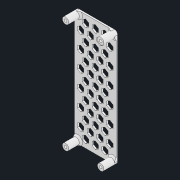
# Autodesk Inventor part: scara-base30
Saved by Autodesk Inventor 2022 (Build 260153000, 153)
## iProperties
Created: 2021-11-06
Part Number: scara-base30
Material: ABS プラスチック
Document SubType Name: Modeling
Designer: Yuta Kage
Density: 1.06 g/cm^3
Appearance: 滑らか - 白
Author: Yuta Kage
Autodesk Inventor part; units mm, degrees
ref_plane "YZ Plane" through (0, 0, 0) normal (1, 0, 0) x (0, 1, 0)
ref_plane "XZ Plane" through (0, 0, 0) normal (0, 1, 0) x (-1, 0, 0)
ref_plane "XY Plane" through (0, 0, 0) normal (0, 0, 1) x (1, 0, 0)
sketch "スケッチ1" plane through (0, 0, 0) normal (0, 0, 1) x (1, 0, 0)
  line L0 (-25.75, -71.75) -> (25.75, -71.75)
  line L1 (25.75, -71.75) -> (25.75, 71.75)
  line L2 (25.75, 71.75) -> (-25.75, 71.75)
  line L3 (-25.75, 71.75) -> (-25.75, -71.75)
  point P0 (0, 0)
  dimension "d0" = 143.5
  dimension "d1" = 51.5
  dimension "d2" = 71.75
  dimension "d3" = 25.75
  constraints: 8 end point, 2 parallel, 1 horizontal, 1 perpendicular
  measures "d0" distance of L2.end L0.start
  measures "d1" distance of L1.end L2.end
  measures "d2" distance from line of point (0, 0) L2
  measures "d3" distance from line of point (0, 0) L3
extrude "押し出し1" add sketch "スケッチ1" along normal blind 2
sketch "スケッチ2" plane through (0, 0, 2) normal (0, 0, 1) x (1, 0, 0)
  line L0 (-12, -57.735) -> (-8, -60.0444)
  line L1 (-8, -60.0444) -> (-8, -64.6632)
  line L2 (-8, -64.6632) -> (-12, -66.9726)
  line L3 (-12, -66.9726) -> (-16, -64.6632)
  line L4 (-16, -64.6632) -> (-16, -60.0444)
  line L5 (-16, -60.0444) -> (-12, -57.735)
  line L6 (-18, -47.3427) -> (-14, -49.6521)
  line L7 (-14, -49.6521) -> (-14, -54.2709)
  line L8 (-14, -54.2709) -> (-18, -56.5803)
  line L9 (-18, -56.5803) -> (-22, -54.2709)
  line L10 (-22, -54.2709) -> (-22, -49.6521)
  line L11 (-22, -49.6521) -> (-18, -47.3427)
  line L12 (-25.75, 71.75) -> (-25.75, -71.75) construction
  line L13 (-25.75, -71.75) -> (25.75, -71.75) projected
  line L14 (-37.6, 0) -> (38.35, 0) construction
  line L15 (0, -104.0432) -> (0, 115.0089) construction
  line L16 (-18, -26.5581) -> (-14, -28.8675)
  line L17 (-22, -28.8675) -> (-18, -26.5581)
  line L18 (-14, -28.8675) -> (-14, -33.4863)
  line L19 (-22, -33.4863) -> (-22, -28.8675)
  line L20 (-14, -33.4863) -> (-18, -35.7957)
  line L21 (-18, -35.7957) -> (-22, -33.4863)
  line L22 (-12, -36.9504) -> (-8, -39.2598)
  line L23 (-16, -39.2598) -> (-12, -36.9504)
  line L24 (-8, -39.2598) -> (-8, -43.8786)
  line L25 (-16, -43.8786) -> (-16, -39.2598)
  line L26 (-8, -43.8786) -> (-12, -46.188)
  line L27 (-12, -46.188) -> (-16, -43.8786)
  line L28 (-6, -47.3427) -> (-2, -49.6521)
  line L29 (-10, -49.6521) -> (-6, -47.3427)
  line L30 (-2, -49.6521) -> (-2, -54.2709)
  line L31 (-10, -54.2709) -> (-10, -49.6521)
  line L32 (-2, -54.2709) -> (-6, -56.5803)
  line L33 (-6, -56.5803) -> (-10, -54.2709)
  line L34 (0, -57.735) -> (4, -60.0444)
  line L35 (-4, -60.0444) -> (0, -57.735)
  line L36 (4, -60.0444) -> (4, -64.6632)
  line L37 (-4, -64.6632) -> (-4, -60.0444)
  line L38 (4, -64.6632) -> (0, -66.9726)
  line L39 (0, -66.9726) -> (-4, -64.6632)
  line L40 (-6, -26.5581) -> (-2, -28.8675)
  line L41 (-10, -28.8675) -> (-6, -26.5581)
  line L42 (-2, -28.8675) -> (-2, -33.4863)
  line L43 (-10, -33.4863) -> (-10, -28.8675)
  line L44 (-2, -33.4863) -> (-6, -35.7957)
  line L45 (-6, -35.7957) -> (-10, -33.4863)
  line L46 (0, -36.9504) -> (4, -39.2598)
  line L47 (-4, -39.2598) -> (0, -36.9504)
  line L48 (4, -39.2598) -> (4, -43.8786)
  line L49 (-4, -43.8786) -> (-4, -39.2598)
  line L50 (4, -43.8786) -> (0, -46.188)
  line L51 (0, -46.188) -> (-4, -43.8786)
  line L52 (-18, -5.7735) -> (-14, -8.0829)
  line L53 (-22, -8.0829) -> (-18, -5.7735)
  line L54 (-14, -8.0829) -> (-14, -12.7017)
  line L55 (-22, -12.7017) -> (-22, -8.0829)
  line L56 (-14, -12.7017) -> (-18, -15.0111)
  line L57 (-18, -15.0111) -> (-22, -12.7017)
  line L58 (-12, -16.1658) -> (-8, -18.4752)
  line L59 (-16, -18.4752) -> (-12, -16.1658)
  line L60 (-8, -18.4752) -> (-8, -23.094)
  line L61 (-16, -23.094) -> (-16, -18.4752)
  line L62 (-8, -23.094) -> (-12, -25.4034)
  line L63 (-12, -25.4034) -> (-16, -23.094)
  line L64 (-6, -5.7735) -> (-2, -8.0829)
  line L65 (-10, -8.0829) -> (-6, -5.7735)
  line L66 (-2, -8.0829) -> (-2, -12.7017)
  line L67 (-10, -12.7017) -> (-10, -8.0829)
  line L68 (-2, -12.7017) -> (-6, -15.0111)
  line L69 (-6, -15.0111) -> (-10, -12.7017)
  line L70 (0, -16.1658) -> (4, -18.4752)
  line L71 (-4, -18.4752) -> (0, -16.1658)
  line L72 (4, -18.4752) -> (4, -23.094)
  line L73 (-4, -23.094) -> (-4, -18.4752)
  line L74 (4, -23.094) -> (0, -25.4034)
  line L75 (0, -25.4034) -> (-4, -23.094)
  line L76 (-18, 15.0111) -> (-14, 12.7017)
  line L77 (-22, 12.7017) -> (-18, 15.0111)
  line L78 (-14, 12.7017) -> (-14, 8.0829)
  line L79 (-22, 8.0829) -> (-22, 12.7017)
  line L80 (-14, 8.0829) -> (-18, 5.7735)
  line L81 (-18, 5.7735) -> (-22, 8.0829)
  line L82 (-12, 4.6188) -> (-8, 2.3094)
  line L83 (-16, 2.3094) -> (-12, 4.6188)
  line L84 (-8, 2.3094) -> (-8, -2.3094)
  line L85 (-16, -2.3094) -> (-16, 2.3094)
  line L86 (-8, -2.3094) -> (-12, -4.6188)
  line L87 (-12, -4.6188) -> (-16, -2.3094)
  line L88 (-6, 15.0111) -> (-2, 12.7017)
  line L89 (-10, 12.7017) -> (-6, 15.0111)
  line L90 (-2, 12.7017) -> (-2, 8.0829)
  line L91 (-10, 8.0829) -> (-10, 12.7017)
  line L92 (-2, 8.0829) -> (-6, 5.7735)
  line L93 (-6, 5.7735) -> (-10, 8.0829)
  line L94 (0, 4.6188) -> (4, 2.3094)
  line L95 (-4, 2.3094) -> (0, 4.6188)
  line L96 (4, 2.3094) -> (4, -2.3094)
  line L97 (-4, -2.3094) -> (-4, 2.3094)
  line L98 (4, -2.3094) -> (0, -4.6188)
  line L99 (0, -4.6188) -> (-4, -2.3094)
  line L100 (-18, 35.7957) -> (-14, 33.4863)
  line L101 (-22, 33.4863) -> (-18, 35.7957)
  line L102 (-14, 33.4863) -> (-14, 28.8675)
  line L103 (-22, 28.8675) -> (-22, 33.4863)
  line L104 (-14, 28.8675) -> (-18, 26.5581)
  line L105 (-18, 26.5581) -> (-22, 28.8675)
  line L106 (-12, 25.4034) -> (-8, 23.094)
  line L107 (-16, 23.094) -> (-12, 25.4034)
  line L108 (-8, 23.094) -> (-8, 18.4752)
  line L109 (-16, 18.4752) -> (-16, 23.094)
  line L110 (-8, 18.4752) -> (-12, 16.1658)
  line L111 (-12, 16.1658) -> (-16, 18.4752)
  line L112 (-6, 35.7957) -> (-2, 33.4863)
  line L113 (-10, 33.4863) -> (-6, 35.7957)
  line L114 (-2, 33.4863) -> (-2, 28.8675)
  line L115 (-10, 28.8675) -> (-10, 33.4863)
  line L116 (-2, 28.8675) -> (-6, 26.5581)
  line L117 (-6, 26.5581) -> (-10, 28.8675)
  line L118 (0, 25.4034) -> (4, 23.094)
  line L119 (-4, 23.094) -> (0, 25.4034)
  line L120 (4, 23.094) -> (4, 18.4752)
  line L121 (-4, 18.4752) -> (-4, 23.094)
  line L122 (4, 18.4752) -> (0, 16.1658)
  line L123 (0, 16.1658) -> (-4, 18.4752)
  line L124 (-18, 56.5803) -> (-14, 54.2709)
  line L125 (-22, 54.2709) -> (-18, 56.5803)
  line L126 (-14, 54.2709) -> (-14, 49.6521)
  line L127 (-22, 49.6521) -> (-22, 54.2709)
  line L128 (-14, 49.6521) -> (-18, 47.3427)
  line L129 (-18, 47.3427) -> (-22, 49.6521)
  line L130 (-12, 46.188) -> (-8, 43.8786)
  line L131 (-16, 43.8786) -> (-12, 46.188)
  line L132 (-8, 43.8786) -> (-8, 39.2598)
  line L133 (-16, 39.2598) -> (-16, 43.8786)
  line L134 (-8, 39.2598) -> (-12, 36.9504)
  line L135 (-12, 36.9504) -> (-16, 39.2598)
  line L136 (-6, 56.5803) -> (-2, 54.2709)
  line L137 (-10, 54.2709) -> (-6, 56.5803)
  line L138 (-2, 54.2709) -> (-2, 49.6521)
  line L139 (-10, 49.6521) -> (-10, 54.2709)
  line L140 (-2, 49.6521) -> (-6, 47.3427)
  line L141 (-6, 47.3427) -> (-10, 49.6521)
  line L142 (0, 46.188) -> (4, 43.8786)
  line L143 (-4, 43.8786) -> (0, 46.188)
  line L144 (4, 43.8786) -> (4, 39.2598)
  line L145 (-4, 39.2598) -> (-4, 43.8786)
  line L146 (4, 39.2598) -> (0, 36.9504)
  line L147 (0, 36.9504) -> (-4, 39.2598)
  line L148 (6, -47.3427) -> (10, -49.6521)
  line L149 (2, -49.6521) -> (6, -47.3427)
  line L150 (10, -49.6521) -> (10, -54.2709)
  line L151 (2, -54.2709) -> (2, -49.6521)
  line L152 (10, -54.2709) -> (6, -56.5803)
  line L153 (6, -56.5803) -> (2, -54.2709)
  line L154 (12, -57.735) -> (16, -60.0444)
  line L155 (8, -60.0444) -> (12, -57.735)
  line L156 (16, -60.0444) -> (16, -64.6632)
  line L157 (8, -64.6632) -> (8, -60.0444)
  line L158 (16, -64.6632) -> (12, -66.9726)
  line L159 (12, -66.9726) -> (8, -64.6632)
  line L160 (6, -26.5581) -> (10, -28.8675)
  line L161 (2, -28.8675) -> (6, -26.5581)
  line L162 (10, -28.8675) -> (10, -33.4863)
  line L163 (2, -33.4863) -> (2, -28.8675)
  line L164 (10, -33.4863) -> (6, -35.7957)
  line L165 (6, -35.7957) -> (2, -33.4863)
  line L166 (12, -36.9504) -> (16, -39.2598)
  line L167 (8, -39.2598) -> (12, -36.9504)
  line L168 (16, -39.2598) -> (16, -43.8786)
  line L169 (8, -43.8786) -> (8, -39.2598)
  line L170 (16, -43.8786) -> (12, -46.188)
  line L171 (12, -46.188) -> (8, -43.8786)
  line L172 (6, -5.7735) -> (10, -8.0829)
  line L173 (2, -8.0829) -> (6, -5.7735)
  line L174 (10, -8.0829) -> (10, -12.7017)
  line L175 (2, -12.7017) -> (2, -8.0829)
  line L176 (10, -12.7017) -> (6, -15.0111)
  line L177 (6, -15.0111) -> (2, -12.7017)
  line L178 (12, -16.1658) -> (16, -18.4752)
  line L179 (8, -18.4752) -> (12, -16.1658)
  line L180 (16, -18.4752) -> (16, -23.094)
  line L181 (8, -23.094) -> (8, -18.4752)
  line L182 (16, -23.094) -> (12, -25.4034)
  line L183 (12, -25.4034) -> (8, -23.094)
  line L184 (6, 15.0111) -> (10, 12.7017)
  line L185 (2, 12.7017) -> (6, 15.0111)
  line L186 (10, 12.7017) -> (10, 8.0829)
  line L187 (2, 8.0829) -> (2, 12.7017)
  line L188 (10, 8.0829) -> (6, 5.7735)
  line L189 (6, 5.7735) -> (2, 8.0829)
  line L190 (12, 4.6188) -> (16, 2.3094)
  line L191 (8, 2.3094) -> (12, 4.6188)
  line L192 (16, 2.3094) -> (16, -2.3094)
  line L193 (8, -2.3094) -> (8, 2.3094)
  line L194 (16, -2.3094) -> (12, -4.6188)
  line L195 (12, -4.6188) -> (8, -2.3094)
  line L196 (6, 35.7957) -> (10, 33.4863)
  line L197 (2, 33.4863) -> (6, 35.7957)
  line L198 (10, 33.4863) -> (10, 28.8675)
  line L199 (2, 28.8675) -> (2, 33.4863)
  line L200 (10, 28.8675) -> (6, 26.5581)
  line L201 (6, 26.5581) -> (2, 28.8675)
  line L202 (12, 25.4034) -> (16, 23.094)
  line L203 (8, 23.094) -> (12, 25.4034)
  line L204 (16, 23.094) -> (16, 18.4752)
  line L205 (8, 18.4752) -> (8, 23.094)
  line L206 (16, 18.4752) -> (12, 16.1658)
  line L207 (12, 16.1658) -> (8, 18.4752)
  line L208 (6, 56.5803) -> (10, 54.2709)
  line L209 (2, 54.2709) -> (6, 56.5803)
  line L210 (10, 54.2709) -> (10, 49.6521)
  line L211 (2, 49.6521) -> (2, 54.2709)
  line L212 (10, 49.6521) -> (6, 47.3427)
  line L213 (6, 47.3427) -> (2, 49.6521)
  line L214 (12, 46.188) -> (16, 43.8786)
  line L215 (8, 43.8786) -> (12, 46.188)
  line L216 (16, 43.8786) -> (16, 39.2598)
  line L217 (8, 39.2598) -> (8, 43.8786)
  line L218 (16, 39.2598) -> (12, 36.9504)
  line L219 (12, 36.9504) -> (8, 39.2598)
  line L220 (18, -47.3427) -> (22, -49.6521)
  line L221 (14, -49.6521) -> (18, -47.3427)
  line L222 (22, -49.6521) -> (22, -54.2709)
  line L223 (14, -54.2709) -> (14, -49.6521)
  line L224 (22, -54.2709) -> (18, -56.5803)
  line L225 (18, -56.5803) -> (14, -54.2709)
  line L226 (24, -57.735) -> (28, -60.0444)
  line L227 (20, -60.0444) -> (24, -57.735)
  line L228 (28, -60.0444) -> (28, -64.6632)
  line L229 (20, -64.6632) -> (20, -60.0444)
  line L230 (28, -64.6632) -> (24, -66.9726)
  line L231 (24, -66.9726) -> (20, -64.6632)
  line L232 (18, -26.5581) -> (22, -28.8675)
  line L233 (14, -28.8675) -> (18, -26.5581)
  line L234 (22, -28.8675) -> (22, -33.4863)
  line L235 (14, -33.4863) -> (14, -28.8675)
  line L236 (22, -33.4863) -> (18, -35.7957)
  line L237 (18, -35.7957) -> (14, -33.4863)
  line L238 (24, -36.9504) -> (28, -39.2598)
  line L239 (20, -39.2598) -> (24, -36.9504)
  line L240 (28, -39.2598) -> (28, -43.8786)
  line L241 (20, -43.8786) -> (20, -39.2598)
  line L242 (28, -43.8786) -> (24, -46.188)
  line L243 (24, -46.188) -> (20, -43.8786)
  line L244 (18, -5.7735) -> (22, -8.0829)
  line L245 (14, -8.0829) -> (18, -5.7735)
  line L246 (22, -8.0829) -> (22, -12.7017)
  line L247 (14, -12.7017) -> (14, -8.0829)
  line L248 (22, -12.7017) -> (18, -15.0111)
  line L249 (18, -15.0111) -> (14, -12.7017)
  line L250 (24, -16.1658) -> (28, -18.4752)
  line L251 (20, -18.4752) -> (24, -16.1658)
  line L252 (28, -18.4752) -> (28, -23.094)
  line L253 (20, -23.094) -> (20, -18.4752)
  line L254 (28, -23.094) -> (24, -25.4034)
  line L255 (24, -25.4034) -> (20, -23.094)
  line L256 (18, 15.0111) -> (22, 12.7017)
  line L257 (14, 12.7017) -> (18, 15.0111)
  line L258 (22, 12.7017) -> (22, 8.0829)
  line L259 (14, 8.0829) -> (14, 12.7017)
  line L260 (22, 8.0829) -> (18, 5.7735)
  line L261 (18, 5.7735) -> (14, 8.0829)
  line L262 (24, 4.6188) -> (28, 2.3094)
  line L263 (20, 2.3094) -> (24, 4.6188)
  line L264 (28, 2.3094) -> (28, -2.3094)
  line L265 (20, -2.3094) -> (20, 2.3094)
  line L266 (28, -2.3094) -> (24, -4.6188)
  line L267 (24, -4.6188) -> (20, -2.3094)
  line L268 (18, 35.7957) -> (22, 33.4863)
  line L269 (14, 33.4863) -> (18, 35.7957)
  line L270 (22, 33.4863) -> (22, 28.8675)
  line L271 (14, 28.8675) -> (14, 33.4863)
  line L272 (22, 28.8675) -> (18, 26.5581)
  line L273 (18, 26.5581) -> (14, 28.8675)
  line L274 (24, 25.4034) -> (28, 23.094)
  line L275 (20, 23.094) -> (24, 25.4034)
  line L276 (28, 23.094) -> (28, 18.4752)
  line L277 (20, 18.4752) -> (20, 23.094)
  line L278 (28, 18.4752) -> (24, 16.1658)
  line L279 (24, 16.1658) -> (20, 18.4752)
  line L280 (18, 56.5803) -> (22, 54.2709)
  line L281 (14, 54.2709) -> (18, 56.5803)
  line L282 (22, 54.2709) -> (22, 49.6521)
  line L283 (14, 49.6521) -> (14, 54.2709)
  line L284 (22, 49.6521) -> (18, 47.3427)
  line L285 (18, 47.3427) -> (14, 49.6521)
  line L286 (24, 46.188) -> (28, 43.8786)
  line L287 (20, 43.8786) -> (24, 46.188)
  line L288 (28, 43.8786) -> (28, 39.2598)
  line L289 (20, 39.2598) -> (20, 43.8786)
  line L290 (28, 39.2598) -> (24, 36.9504)
  line L291 (24, 36.9504) -> (20, 39.2598)
  line L292 (-18, 77.3649) -> (-14, 75.0555)
  line L293 (-22, 75.0555) -> (-18, 77.3649)
  line L294 (-14, 75.0555) -> (-14, 70.4367)
  line L295 (-22, 70.4367) -> (-22, 75.0555)
  line L296 (-14, 70.4367) -> (-18, 68.1273)
  line L297 (-18, 68.1273) -> (-22, 70.4367)
  line L298 (-12, 66.9726) -> (-8, 64.6632)
  line L299 (-16, 64.6632) -> (-12, 66.9726)
  line L300 (-8, 64.6632) -> (-8, 60.0444)
  line L301 (-16, 60.0444) -> (-16, 64.6632)
  line L302 (-8, 60.0444) -> (-12, 57.735)
  line L303 (-12, 57.735) -> (-16, 60.0444)
  line L304 (-6, 77.3649) -> (-2, 75.0555)
  line L305 (-10, 75.0555) -> (-6, 77.3649)
  line L306 (-2, 75.0555) -> (-2, 70.4367)
  line L307 (-10, 70.4367) -> (-10, 75.0555)
  line L308 (-2, 70.4367) -> (-6, 68.1273)
  line L309 (-6, 68.1273) -> (-10, 70.4367)
  line L310 (0, 66.9726) -> (4, 64.6632)
  line L311 (-4, 64.6632) -> (0, 66.9726)
  line L312 (4, 64.6632) -> (4, 60.0444)
  line L313 (-4, 60.0444) -> (-4, 64.6632)
  line L314 (4, 60.0444) -> (0, 57.735)
  line L315 (0, 57.735) -> (-4, 60.0444)
  line L316 (6, 77.3649) -> (10, 75.0555)
  line L317 (2, 75.0555) -> (6, 77.3649)
  line L318 (10, 75.0555) -> (10, 70.4367)
  line L319 (2, 70.4367) -> (2, 75.0555)
  line L320 (10, 70.4367) -> (6, 68.1273)
  line L321 (6, 68.1273) -> (2, 70.4367)
  line L322 (12, 66.9726) -> (16, 64.6632)
  line L323 (8, 64.6632) -> (12, 66.9726)
  line L324 (16, 64.6632) -> (16, 60.0444)
  line L325 (8, 60.0444) -> (8, 64.6632)
  line L326 (16, 60.0444) -> (12, 57.735)
  line L327 (12, 57.735) -> (8, 60.0444)
  line L328 (18, 77.3649) -> (22, 75.0555)
  line L329 (14, 75.0555) -> (18, 77.3649)
  line L330 (22, 75.0555) -> (22, 70.4367)
  line L331 (14, 70.4367) -> (14, 75.0555)
  line L332 (22, 70.4367) -> (18, 68.1273)
  line L333 (18, 68.1273) -> (14, 70.4367)
  line L334 (24, 66.9726) -> (28, 64.6632)
  line L335 (20, 64.6632) -> (24, 66.9726)
  line L336 (28, 64.6632) -> (28, 60.0444)
  line L337 (20, 60.0444) -> (20, 64.6632)
  line L338 (28, 60.0444) -> (24, 57.735)
  line L339 (24, 57.735) -> (20, 60.0444)
  point P0 (-12, -62.3538)
  point P1 (-18, -51.9615)
  point P2 (-12, -41.5692)
  point P3 (-18, -31.1769)
  point P4 (-25.75, -50.9654)
  point P5 (0, -62.3538)
  point P6 (-6, -51.9615)
  point P7 (-13.75, -71.75)
  point P8 (0, -41.5692)
  point P9 (-6, -31.1769)
  point P10 (-13.75, -50.9654)
  point P11 (-12, -20.7846)
  point P12 (-18, -10.3923)
  point P13 (-25.75, -30.1808)
  point P14 (0, -20.7846)
  point P15 (-6, -10.3923)
  point P16 (-13.75, -30.1808)
  point P17 (-12, 0)
  point P18 (-18, 10.3923)
  point P19 (-25.75, -9.3962)
  point P20 (0, 0)
  point P21 (-6, 10.3923)
  point P22 (-13.75, -9.3962)
  point P23 (-12, 20.7846)
  point P24 (-18, 31.1769)
  point P25 (-25.75, 11.3884)
  point P26 (0, 20.7846)
  point P27 (-6, 31.1769)
  point P28 (-13.75, 11.3884)
  point P29 (-12, 41.5692)
  point P30 (-18, 51.9615)
  point P31 (-25.75, 32.173)
  point P32 (0, 41.5692)
  point P33 (-6, 51.9615)
  point P34 (-13.75, 32.173)
  point P35 (12, -62.3538)
  point P36 (6, -51.9615)
  point P37 (-1.75, -71.75)
  point P38 (12, -41.5692)
  point P39 (6, -31.1769)
  point P40 (-1.75, -50.9654)
  point P41 (12, -20.7846)
  point P42 (6, -10.3923)
  point P43 (-1.75, -30.1808)
  point P44 (12, 0)
  point P45 (6, 10.3923)
  point P46 (-1.75, -9.3962)
  point P47 (12, 20.7846)
  point P48 (6, 31.1769)
  point P49 (-1.75, 11.3884)
  point P50 (12, 41.5692)
  point P51 (6, 51.9615)
  point P52 (-1.75, 32.173)
  point P53 (24, -62.3538)
  point P54 (18, -51.9615)
  point P55 (10.25, -71.75)
  point P56 (24, -41.5692)
  point P57 (18, -31.1769)
  point P58 (10.25, -50.9654)
  point P59 (24, -20.7846)
  point P60 (18, -10.3923)
  point P61 (10.25, -30.1808)
  point P62 (24, 0)
  point P63 (18, 10.3923)
  point P64 (10.25, -9.3962)
  point P65 (24, 20.7846)
  point P66 (18, 31.1769)
  point P67 (10.25, 11.3884)
  point P68 (24, 41.5692)
  point P69 (18, 51.9615)
  point P70 (10.25, 32.173)
  point P71 (-12, 62.3538)
  point P72 (-18, 72.7461)
  point P73 (-25.75, 52.9577)
  point P74 (0, 62.3538)
  point P75 (-6, 72.7461)
  point P76 (-13.75, 52.9577)
  point P77 (12, 62.3538)
  point P78 (6, 72.7461)
  point P79 (-1.75, 52.9577)
  point P80 (24, 62.3538)
  point P81 (18, 72.7461)
  point P82 (10.25, 52.9577)
  point P83 (0, 0)
  dimension "d6" = 8
  dimension "d15" = 8
  dimension "d18" = 20.7846
  dimension "d21" = 12
  dimension "d24" = 10.3923
  dimension "d37" = 4
  dimension "d38" = 4
  constraints: 672 end point, 1 coincident, 1 horizontal, 1 parallel, 1 vertical, 755 other
  measures "d6" distance between parallel lines of L1 L4
  measures "d15" distance between parallel lines of L10 L7
  measures "d18" distance of point (-12, -62.354) point (-12, -41.569)
  measures "d21" distance of point (-12, -62.354) point (0, -62.354)
  measures "d24" vertical distance of point (-12, -62.354) point (-18, -51.962)
  measures "d37" distance between parallel lines of L5 L8
  measures "d38" distance between parallel lines of L0 L33
extrude "押し出し2" cut sketch "スケッチ2" against normal through all contours L0 L1 L2 L3 L4 L5 | L6 L7 L8 L9 L10 L11 | L16 L18 L20 L21 L19 L17 | L22 L24 L26 L27 L25 L23 | L28 L30 L32 L33 L31 L29 | L34 L36 L38 L39 L37 L35 | L40 L42 L44 L45 L43 L41 | L46 L48 L50 L51 L49 L47 | L52 L54 L56 L57 L55 L53 | L58 L60 L62 L63 L61 L59 | L64 L66 L68 L69 L67 L65 | L70 L72 L74 L75 L73 L71 | L76 L78 L80 L81 L79 L77 | L82 L84 L86 L87 L85 L83 | L88 L90 L92 L93 L91 L89 | L94 L96 L98 L99 L97 L95 | L100 L102 L104 L105 L103 L101 | L106 L108 L110 L111 L109 L107 | L112 L114 L116 L117 L115 L113 | L118 L120 L122 L123 L121 L119 | L124 L126 L128 L129 L127 L125 | L130 L132 L134 L135 L133 L131 | L136 L138 L140 L141 L139 L137 | L142 L144 L146 L147 L145 L143 | L148 L150 L152 L153 L151 L149 | L154 L156 L158 L159 L157 L155 | L160 L162 L164 L165 L163 L161 | L166 L168 L170 L171 L169 L167 | L172 L174 L176 L177 L175 L173 | L178 L180 L182 L183 L181 L179 | L184 L186 L188 L189 L187 L185 | L190 L192 L194 L195 L193 L191 | L196 L198 L200 L201 L199 L197 | L202 L204 L206 L207 L205 L203 | L208 L210 L212 L213 L211 L209 | L214 L216 L218 L219 L217 L215 | L220 L222 L224 L225 L223 L221 | L232 L234 L236 L237 L235 L233 | L244 L246 L248 L249 L247 L245 | L256 L258 L260 L261 L259 L257 | L268 L270 L272 L273 L271 L269 | L280 L282 L284 L285 L283 L281 | L298 L300 L302 L303 L301 L299 | L310 L312 L314 L315 L313 L311 | L322 L324 L326 L327 L325 L323
sketch "スケッチ3" plane through (0, 0, 0) normal (0, 0, 1) x (1, 0, 0)
  line L0 (-21.75, -67.75) -> (21.75, -67.75) construction
  line L1 (21.75, -67.75) -> (21.75, 67.75) construction
  line L2 (21.75, 67.75) -> (-21.75, 67.75) construction
  line L3 (-21.75, 67.75) -> (-21.75, -67.75) construction
  line L4 (-21.75, -67.75) -> (21.75, 67.75) construction
  line L5 (21.75, -67.75) -> (-21.75, 67.75) construction
  line L6 (-17.75, 63.75) -> (-25.75, 63.75)
  line L7 (-25.75, 63.75) -> (-25.75, 71.75)
  line L8 (-25.75, 71.75) -> (-17.75, 71.75)
  line L9 (-17.75, 71.75) -> (-17.75, 63.75)
  line L10 (-17.75, 63.75) -> (-25.75, 71.75) construction
  line L11 (-25.75, 63.75) -> (-17.75, 71.75) construction
  line L12 (25.75, 63.75) -> (17.75, 63.75)
  line L13 (17.75, 63.75) -> (17.75, 71.75)
  line L14 (17.75, 71.75) -> (25.75, 71.75)
  line L15 (25.75, 71.75) -> (25.75, 63.75)
  line L16 (25.75, 63.75) -> (17.75, 71.75) construction
  line L17 (17.75, 63.75) -> (25.75, 71.75) construction
  line L18 (-17.75, -71.75) -> (-25.75, -71.75)
  line L19 (-25.75, -71.75) -> (-25.75, -63.75)
  line L20 (-25.75, -63.75) -> (-17.75, -63.75)
  line L21 (-17.75, -63.75) -> (-17.75, -71.75)
  line L22 (-17.75, -71.75) -> (-25.75, -63.75) construction
  line L23 (-25.75, -71.75) -> (-17.75, -63.75) construction
  line L24 (25.75, -71.75) -> (17.75, -71.75)
  line L25 (17.75, -71.75) -> (17.75, -63.75)
  line L26 (17.75, -63.75) -> (25.75, -63.75)
  line L27 (25.75, -63.75) -> (25.75, -71.75)
  line L28 (25.75, -71.75) -> (17.75, -63.75) construction
  line L29 (17.75, -71.75) -> (25.75, -63.75) construction
  point P0 (0, 0)
  dimension "d28" = 43.5
  dimension "d29" = 135.5
  dimension "d42" = 43.5
  dimension "d45" = 135.5
  constraints: 60 end point, 10 midpoint, 4 coincident, 4 parallel, 3 horizontal, 2 perpendicular, 1 vertical, 33 other
  measures "d28" distance of L2.end L1.end
  measures "d29" distance of L1.end L0.end
  measures "d42" distance of L2.end point (21.75, 67.75)
  measures "d45" distance of L2.end point (-21.75, -67.75)
extrude "押し出し3" add sketch "スケッチ3" along normal blind 17
hole "穴2" at (-21.75, 67.75, 0) at (21.75, 67.75, 0) at (21.75, -67.75, 0) at (-21.75, -67.75, 0) direction (0, 0, 1) diameter 3.4 end through all clearance for "Flat Head Machine Screw" size "M3" standard "Ansi Metric M Profile"
fillet "フィレット2" radius 4 4 edges at (-25.75, 71.75, 8.5) (25.75, 71.75, 8.5) (-25.75, -71.75, 8.5) (25.75, -71.75, 8.5)
fillet "フィレット3" radius 4 12 edges at (-17.75, -71.75, 9.5) (17.75, -71.75, 9.5) (17.75, -63.75, 9.5) (25.75, -63.75, 9.5) (-17.75, 71.75, 9.5) (-17.75, 63.75, 9.5) (-25.75, 63.75, 9.5) (-25.75, -63.75, 9.5) (-17.75, -63.75, 9.5) (25.75, 63.75, 9.5) (17.75, 63.75, 9.5) (17.75, 71.75, 9.5)
chamfer "面取り1" distance 2 angle 45 20 edges at (18.9215, -70.5785, 2) (17.75, -67.75, 2) (18.9215, -64.9215, 2) (21.75, -63.75, 2) (24.5785, -64.9215, 2) (-18.9215, -70.5785, 2) (-17.75, -67.75, 2) (-18.9215, -64.9215, 2) (-21.75, -63.75, 2) (-24.5785, -64.9215, 2) (-24.5785, 64.9215, 2) (-21.75, 63.75, 2) (-18.9215, 64.9215, 2) (-17.75, 67.75, 2) (-18.9215, 70.5785, 2) (24.5785, 64.9215, 2) (21.75, 63.75, 2) (18.9215, 70.5785, 2) (18.9215, 64.9215, 2) (17.75, 67.75, 2)
equation "\"d2\" = 0.5 * d0"
equation "\"d3\" = 0.5 * d1"
equation "\"d15\" = d6"
equation "\"d18\" = 2 * d24"
equation "\"d21\" = 3 * d37"
equation "\"d37\" = 0.5 * d6"
equation "\"d38\" = 0.5 * d6"
equation "\"d42\" = d28"
equation "\"d45\" = d29"
